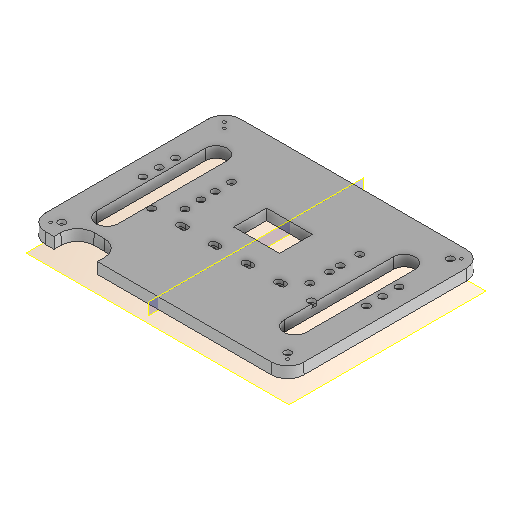
# Autodesk Inventor part: 60_Planktoscope_MicroscopeHolder_Bottom_v0
Saved by Autodesk Inventor 2024.1 (Build 281209000, 209)
## iProperties
Created: 2024-06-29
Part Number: 60_Planktoscope_MicroscopeHolder_Bottom_v0
Material: Generisch
Document SubType Name: Modeling
Designer: diederichbenedict
Density: 1 g/cm^3
Appearance: Vorgabe
Vendor: openUC2
Mass: 350.769 g
Surface Area: 894.112 cm^2
Volume: 350.769 cm^3
Author: diederichbenedict
Autodesk Inventor part; units mm, degrees
ref_plane "YZ Plane" through (0, 0, 0) normal (1, 0, 0) x (0, 1, 0)
ref_plane "XZ Plane" through (0, 0, 0) normal (0, 1, 0) x (-1, 0, 0)
ref_plane "XY Plane" through (0, 0, 0) normal (0, 0, 1) x (1, 0, 0)
ref_plane "Arbeitsebene1" through (0, -238.9229, -15) normal (0, 0, 1) x (1, 0, 0)
sketch "Skizze1" plane through (0, -238.9229, 0) normal (0, 0, 1) x (1, 0, 0)
  line L0 (-108.9123, -85.8768) -> (-108, -84.9645) construction
  line L1 (-108, -84.9645) -> (-105.5687, -87.3957) construction
  arc A0 (-105.5687, -87.3957) -> (-101.5, -88) centre (-101.5, -74) ccw construction
  line L2 (-101.5, -88) -> (-95.5, -88) construction
  line L3 (-95.5, -88) -> (-95.5, -75) construction
  arc A1 (-88.5, -68) -> (-95.5, -75) centre (-88.5, -75) ccw construction
  line L4 (-88.5, -68) -> (-62.5, -68) construction
  arc A2 (-55.5, -75) -> (-62.5, -68) centre (-62.5, -75) ccw construction
  line L5 (-55.5, -75) -> (-55.5, -88) construction
  line L6 (-55.5, -88) -> (101.7625, -88) construction
  arc A3 (101.7625, -88) -> (115.5, -74) centre (101.5, -74.0025) ccw construction
  line L7 (115.5, -74) -> (115.5, 74) construction
  arc A4 (115.5, 74) -> (101.7625, 88) centre (101.5, 74.0025) ccw construction
  line L8 (101.7625, 88) -> (-101.5, 88) construction
  arc A5 (-101.5, 88) -> (-115.5, 74) centre (-101.5, 74) ccw construction
  line L9 (-115.5, 74) -> (-115.5, -74) construction
  arc A6 (-115.5, -74) -> (-108.9123, -85.8768) centre (-101.5, -74) ccw construction
  line L10 (101.6984, -82) -> (101.3016, -82) construction
  arc A7 (101.3016, -82) -> (101.6984, -82) centre (101.5, -74.0025) ccw construction
  line L11 (95.5, 73) -> (95.5, 82) construction
  arc A8 (95.5, 73) -> (100.5, 68) centre (100.5, 73) ccw construction
  line L12 (109.5, 68) -> (100.5, 68) construction
  line L13 (109.5, 68) -> (109.5, -68) construction
  line L14 (100.5, -68) -> (109.5, -68) construction
  arc A9 (100.5, -68) -> (95.5, -73) centre (100.5, -73) ccw construction
  line L15 (95.5, -82) -> (95.5, -73) construction
  line L16 (95.5, -82) -> (-49.5, -82) construction
  line L17 (-49.5, -82) -> (-49.5, -75) construction
  arc A10 (-49.5, -75) -> (-62.5, -62) centre (-62.5, -75) ccw construction
  line L18 (-62.5, -62) -> (-88.5, -62) construction
  arc A11 (-88.5, -62) -> (-99.5163, -68.0977) centre (-88.5, -75) ccw construction
  arc A12 (-99.5163, -68.0977) -> (-100.5, -68) centre (-100.5, -73) ccw construction
  line L19 (-109.5, -68) -> (-100.5, -68) construction
  line L20 (-109.5, -68) -> (-109.5, 68) construction
  line L21 (-100.5, 68) -> (-109.5, 68) construction
  arc A13 (-100.5, 68) -> (-95.5, 73) centre (-100.5, 73) ccw construction
  line L22 (-95.5, 82) -> (-95.5, 73) construction
  line L23 (-95.5, 82) -> (95.5, 82) construction
  arc A14 (101.6984, 82) -> (101.3016, 82) centre (101.5, 74.0025) ccw construction
  line L24 (101.3016, 82) -> (101.6984, 82) construction
  line L25 (111.5331, 80.5) -> (107.9975, 76.9645) construction
  line L26 (107.9975, 76.9645) -> (104.462, 80.5) construction
  line L27 (104.462, 80.5) -> (107.9975, 84.0355) construction
  line L28 (107.9975, 84.0355) -> (111.5331, 80.5) construction
  line L29 (108, -84.0355) -> (104.4645, -80.5) construction
  line L30 (104.4645, -80.5) -> (108, -76.9645) construction
  line L31 (108, -76.9645) -> (111.5355, -80.5) construction
  line L32 (111.5355, -80.5) -> (108, -84.0355) construction
  line L33 (-108, 76.9645) -> (-111.5355, 80.5) construction
  line L34 (-111.5355, 80.5) -> (-108, 84.0355) construction
  line L35 (-108, 84.0355) -> (-104.4645, 80.5) construction
  line L36 (-104.4645, 80.5) -> (-108, 76.9645) construction
  circle A15 centre (58.5, 18.7) radius 1.4 projected
  circle A16 centre (58.5, 36.552) radius 1.4 projected
  circle A17 centre (-57.5, 20.252) radius 1.4 projected
  circle A18 centre (-57.5, 35) radius 1.4 projected
  line L37 (-60.5, 13.7) -> (-60.5, 38) construction
  line L38 (61.5, 13.7) -> (-60.5, 13.7) construction
  line L39 (61.5, 38) -> (61.5, 13.7) construction
  line L40 (61.5, 38) -> (-60.5, 38) construction
  circle A19 centre (58.5, 8.7) radius 1.4 projected
  circle A20 centre (58.5, -9.152) radius 1.4 projected
  circle A21 centre (-57.5, 7.148) radius 1.4 projected
  circle A22 centre (-57.5, -7.6) radius 1.4 projected
  line L41 (-60.5, 13.7) -> (-60.5, -10.6) construction
  line L42 (61.5, -10.6) -> (-60.5, -10.6) construction
  line L43 (61.5, -10.6) -> (61.5, 13.7) construction
  line L44 (61.5, 13.7) -> (-60.5, 13.7) construction
  line L45 (-103.5, 89.5) -> (103.5, 89.5)
  line L46 (118.5, 74.5) -> (118.5, -74.5)
  line L47 (103.5, -89.5) -> (-103.5, -89.5)
  line L48 (-118.5, -74.5) -> (-118.5, 74.5)
  arc A23 (-118.5, -74.5) -> (-103.5, -89.5) centre (-103.5, -74.5) ccw
  arc A24 (-103.5, 89.5) -> (-118.5, 74.5) centre (-103.5, 74.5) ccw
  arc A25 (118.5, 74.5) -> (103.5, 89.5) centre (103.5, 74.5) ccw
  arc A26 (103.5, -89.5) -> (118.5, -74.5) centre (103.5, -74.5) ccw
  line L49 (-95.5, -88) -> (-56.1, -88)
  line L50 (-56.1, -88) -> (-56.1, -83)
  line L51 (-71.1, -68) -> (-80.5, -68)
  line L52 (-95.5, -83) -> (-95.5, -88)
  arc A27 (-80.5, -68) -> (-95.5, -83) centre (-80.5, -83) ccw
  arc A28 (-56.1, -83) -> (-71.1, -68) centre (-71.1, -83) ccw
  line L53 (-95.5, -88) -> (-56.1, -88)
  line L54 (-56.1, -88) -> (-56.1, -89.5)
  line L55 (-56.1, -89.5) -> (-95.5, -89.5)
  line L56 (-95.5, -89.5) -> (-95.5, -88)
  point P0 (0, 238.9229)
  point P1 (-103.5567, -87.8481)
  point P2 (-95.5, -87.3481)
  point P3 (-56.1, -87.3481)
  point P4 (-56.1, -88)
  dimension "d0" = 3
  dimension "d1" = 3
  dimension "d4" = 15
  dimension "d5" = 15
  dimension "d42" = 1.5
  dimension "d43" = 1.5
  constraints: 24 end point, 13 point on circle, 12 tangent, 6 centre point, 6 parallel, 4 equal radius, 3 horizontal, 3 perpendicular, 1 point on line
  measures "d0" distance between parallel lines of L48 L9
  measures "d1" distance between parallel lines of L7 L46
  measures "d4" radius of A23
  measures "d5" radius of A27
  measures "d42" distance between parallel lines of L47 L49
  measures "d43" distance between parallel lines of L45 L8
extrude "Extrusion1" add sketch "Skizze1" along normal blind 10 draft -1 contours L45 A25 L46 A26 L47 L54 L50 A28 L51 A27 L52 L56 A23 L48 A24
sketch "Skizze3" plane through (0, -238.9229, 10) normal (0, 0, 1) x (1, 0, 0)
  line L0 (118.3254, 74.5) -> (118.3254, -74.5) projected
  arc A0 (118.3254, 74.5) -> (103.5, 89.3254) centre (103.5, 74.5) ccw projected
  line L1 (-103.5, 89.3254) -> (103.5, 89.3254) projected
  arc A1 (-103.5, 89.3254) -> (-118.3254, 74.5) centre (-103.5, 74.5) ccw projected
  line L2 (-118.3254, -74.5) -> (-118.3254, 74.5) projected
  arc A2 (-118.3254, -74.5) -> (-103.5, -89.3254) centre (-103.5, -74.5) ccw projected
  line L3 (-95.6746, -89.3254) -> (-103.5, -89.3254) projected
  line L4 (-95.6746, -83) -> (-95.6746, -89.3254) projected
  arc A3 (-80.5, -67.8254) -> (-95.6746, -83) centre (-80.5, -83) ccw projected
  line L5 (-71.1, -67.8254) -> (-80.5, -67.8254) projected
  arc A4 (-55.9254, -83) -> (-71.1, -67.8254) centre (-71.1, -83) ccw projected
  line L6 (-55.9254, -89.3254) -> (-55.9254, -83) projected
  arc A5 (103.5, -89.3254) -> (118.3254, -74.5) centre (103.5, -74.5) ccw projected
  circle A6 centre (58.5, 18.7) radius 1.5746 projected
  circle A7 centre (58.5, 36.552) radius 1.5746 projected
  circle A8 centre (-57.5, 20.252) radius 1.5746 projected
  circle A9 centre (-57.5, 35) radius 1.5746 projected
  circle A10 centre (58.5, 8.7) radius 1.5746 projected
  circle A11 centre (58.5, -9.152) radius 1.5746 projected
  circle A12 centre (-57.5, 7.148) radius 1.5746 projected
  circle A13 centre (-57.5, -7.6) radius 1.5746 projected
  line L7 (103.5, -89.3254) -> (-55.9254, -89.3254) projected
  line L8 (103.5, -74.5) -> (-103.5, -74.5)
  line L9 (-103.5, -74.5) -> (-103.5, 74.5)
  line L10 (-103.5, 74.5) -> (103.5, 74.5)
  line L11 (103.5, 74.5) -> (103.5, -74.5)
  line L12 (-108.5, -79.5) -> (108.5, -79.5)
  line L13 (108.5, -79.5) -> (108.5, 79.5)
  line L14 (108.5, 79.5) -> (-108.5, 79.5)
  line L15 (-108.5, 79.5) -> (-108.5, -79.5)
  point P0 (0, 238.9229)
  dimension "d56" = 5
  constraints: 16 end point, 4 parallel, 2 perpendicular, 1 horizontal, 3 other
  measures "d56" distance between parallel lines of L8 L12
hole "Bohrung1" at (-103.5, -164.4229, 10) at (-103.5, -313.4229, 10) at (103.5, -313.4229, 10) at (103.5, -164.4229, 10) at (108.5, -159.4229, 10) at (108.5, -318.4229, 10) at (-108.5, -159.4229, 10) at (-108.5, -318.4229, 10) direction (0, 0, -1) diameter 2.8 end through all
sketch "Skizze4" plane through (0, -238.9229, 10) normal (0, 0, 1) x (1, 0, 0)
  line L0 (-2.75, 38) -> (-2.75, 23.7) projected
  line L1 (-6.0553, 13.7) -> (-6.0553, 30)
  line L2 (20.9, 30.6837) -> (20.9, 6.6837) projected
  line L3 (20.9, 30.6837) -> (-20.9567, 30.6837)
  line L4 (-20.9567, 30.6837) -> (-20.9567, 0.5738)
  line L5 (-20.9567, 0.5738) -> (20.9, 0.5738)
  line L6 (20.9, 0.5738) -> (20.9, 30.6837)
  circle A0 centre (-57.5, 7.148) radius 1.4 projected
  circle A1 centre (-57.5, -10.7039) radius 1.4 projected
  circle A2 centre (58.5, 5.5961) radius 1.4 projected
  circle A3 centre (58.5, -9.152) radius 1.4 projected
  line L7 (-1.5, 2.2357) -> (-1.5, 12.148) projected
  line L8 (-19.5, 2.2357) -> (-1.5, 2.2357) projected
  line L9 (-19.5, 12.148) -> (-19.5, 2.2357) projected
  line L10 (-19.5, 12.148) -> (-60.5, 12.148) projected
  line L11 (-60.5, 12.148) -> (-60.5, -12.152) projected
  line L12 (61.5, -12.152) -> (-60.5, -12.152) projected
  line L13 (61.5, -12.152) -> (61.5, 12.148) projected
  line L14 (61.5, 12.148) -> (-1.5, 12.148) projected
  point P0 (0, 238.9229)
  constraints: 10 end point, 2 parallel, 1 horizontal, 1 perpendicular, 1 vertical, 2 other
extrude "Extrusion3" cut sketch "Skizze4" against normal through all contours L2 L14 L7 L8 L9 L10 L4 L3 | L2 L6 L5 L4 L10 L9 L8 L7 L14
sketch "Skizze5" plane through (0, -238.9229, 10) normal (0, 0, 1) x (1, 0, 0)
  line L0 (-20.9567, 30.6837) -> (20.9, 30.6837) projected
  line L1 (20.9, 30.6837) -> (20.9, 0.5738) projected
  line L2 (20.9, 0.5738) -> (-20.9567, 0.5738) projected
  line L3 (-20.9567, 0.5738) -> (-20.9567, 30.6837) projected
  circle A0 centre (103.5, 74.5) radius 1.4 projected
  circle A1 centre (103.5, -74.5) radius 1.4 projected
  circle A2 centre (-103.5, -74.5) radius 1.4 projected
  circle A3 centre (-103.5, 74.5) radius 1.4 projected
  line L4 (118.3254, 74.5) -> (118.3254, -74.5) projected
  arc A4 (118.3254, 74.5) -> (103.5, 89.3254) centre (103.5, 74.5) ccw projected
  line L5 (-103.5, 89.3254) -> (103.5, 89.3254) projected
  arc A5 (-103.5, 89.3254) -> (-118.3254, 74.5) centre (-103.5, 74.5) ccw projected
  line L6 (-118.3254, -74.5) -> (-118.3254, 74.5) projected
  arc A6 (-118.3254, -74.5) -> (-103.5, -89.3254) centre (-103.5, -74.5) ccw projected
  line L7 (-95.6746, -89.3254) -> (-103.5, -89.3254) projected
  line L8 (-95.6746, -83) -> (-95.6746, -89.3254) projected
  arc A7 (-80.5, -67.8254) -> (-95.6746, -83) centre (-80.5, -83) ccw projected
  line L9 (-71.1, -67.8254) -> (-80.5, -67.8254) projected
  arc A8 (-55.9254, -83) -> (-71.1, -67.8254) centre (-71.1, -83) ccw projected
  line L10 (-55.9254, -89.3254) -> (-55.9254, -83) projected
  arc A9 (103.5, -89.3254) -> (118.3254, -74.5) centre (103.5, -74.5) ccw projected
  circle A10 centre (58.5, 18.7) radius 1.5746 projected
  circle A11 centre (58.5, 36.552) radius 1.5746 projected
  circle A12 centre (-57.5, 20.252) radius 1.5746 projected
  circle A13 centre (-57.5, 35) radius 1.5746 projected
  circle A14 centre (58.5, 8.7) radius 1.5746 projected
  circle A15 centre (58.5, -9.152) radius 1.5746 projected
  circle A16 centre (-57.5, 7.148) radius 1.5746 projected
  circle A17 centre (-57.5, -7.6) radius 1.5746 projected
  line L11 (-73.1917, -22.4328) -> (70.9104, -22.4328)
  line L12 (102.338, 36.5746) -> (102.338, -9.1746)
  line L13 (103.5, -89.3254) -> (-55.9254, -89.3254) projected
  point P0 (0, 238.9229)
  point P1 (-43.1917, -22.4328)
  point P2 (-13.1917, -22.4328)
  point P3 (16.8083, -22.4328)
  point P4 (46.8083, -22.4328)
  point P5 (102.338, 13.7)
  point P6 (102.338, -1.3)
  point P7 (102.338, 28.7)
  point P8 (102.338, 13.7)
  dimension "d21" = 30
  dimension "d36" = 15
  dimension "d39" = 15
  constraints: 4 end point, 3 vertical, 2 horizontal, 1 coincident, 1 midpoint, 7 other
  measures "d21" distance of point (-73.192, -22.433) point (-43.192, -22.433)
  measures "d36" distance of point (102.338, 13.7) point (102.338, -1.3)
  measures "d39" distance of point (102.338, 13.7) point (102.338, 28.7)
hole "Bohrung2" at (-73.1917, -261.3557, 10) at (-43.1917, -261.3557, 10) at (-13.1917, -261.3557, 10) at (16.8083, -261.3557, 10) at (46.8083, -261.3557, 10) at (102.338, -240.2229, 10) at (102.338, -225.2229, 10) at (102.338, -210.2229, 10) direction (0, 0, -1) diameter 2.8 end through all
ref_plane "Arbeitsebene2" through (0, -313.4229, 6788.8605) normal (-1, 0, 0) x (0, -1, 0)
mirror "Spiegeln1" about plane through (0, -313.4229, 6788.8605) normal (-1, 0, 0) of "Bohrung2", "Extrusion3", "Bohrung1"
sketch "Skizze6" plane through (0, -238.9229, 10) normal (0, 0, 1) x (1, 0, 0)
  line L0 (20.9567, 0.5738) -> (-20.9567, 0.5738) projected
  line L1 (-20.9567, 0.5738) -> (-20.9567, 30.6837) projected
  line L2 (-20.9567, 30.6837) -> (20.9567, 30.6837) projected
  line L3 (20.9567, 30.6837) -> (20.9567, 0.5738) projected
  circle A0 centre (-102.338, 13.7) radius 1.4 projected
  circle A1 centre (-102.338, -1.3) radius 1.4 projected
  circle A2 centre (-46.8083, -22.4328) radius 1.4 projected
  circle A3 centre (-16.8083, -22.4328) radius 1.4 projected
  circle A4 centre (13.1917, -22.4328) radius 1.4 projected
  circle A5 centre (43.1917, -22.4328) radius 1.4 projected
  circle A6 centre (73.1917, -22.4328) radius 1.4 projected
  circle A7 centre (-102.338, 28.7) radius 1.4 projected
  circle A8 centre (102.338, 28.7) radius 1.4 projected
  circle A9 centre (102.338, 13.7) radius 1.4 projected
  circle A10 centre (102.338, -1.3) radius 1.4 projected
  circle A11 centre (46.8083, -22.4328) radius 1.4 projected
  circle A12 centre (16.8083, -22.4328) radius 1.4 projected
  circle A13 centre (-13.1917, -22.4328) radius 1.4 projected
  circle A14 centre (-43.1917, -22.4328) radius 1.4 projected
  circle A15 centre (-73.1917, -22.4328) radius 1.4 projected
  circle A16 centre (103.5, 74.5) radius 1.4 projected
  circle A17 centre (103.5, -74.5) radius 1.4 projected
  circle A18 centre (-103.5, -74.5) radius 1.4 projected
  circle A19 centre (-103.5, 74.5) radius 1.4 projected
  circle A20 centre (-57.5, -7.6) radius 1.5746 projected
  circle A21 centre (-57.5, 7.148) radius 1.5746 projected
  circle A22 centre (58.5, -9.152) radius 1.5746 projected
  circle A23 centre (58.5, 8.7) radius 1.5746 projected
  circle A24 centre (-57.5, 35) radius 1.5746 projected
  circle A25 centre (-57.5, 20.252) radius 1.5746 projected
  circle A26 centre (58.5, 36.552) radius 1.5746 projected
  circle A27 centre (58.5, 18.7) radius 1.5746 projected
  line L4 (118.3254, 74.5) -> (118.3254, -74.5) projected
  arc A28 (118.3254, 74.5) -> (103.5, 89.3254) centre (103.5, 74.5) ccw projected
  line L5 (-103.5, 89.3254) -> (103.5, 89.3254) projected
  arc A29 (-103.5, 89.3254) -> (-118.3254, 74.5) centre (-103.5, 74.5) ccw projected
  line L6 (-118.3254, -74.5) -> (-118.3254, 74.5) projected
  arc A30 (-118.3254, -74.5) -> (-103.5, -89.3254) centre (-103.5, -74.5) ccw projected
  line L7 (-95.6746, -89.3254) -> (-103.5, -89.3254) projected
  line L8 (-95.6746, -83) -> (-95.6746, -89.3254) projected
  arc A31 (-80.5, -67.8254) -> (-95.6746, -83) centre (-80.5, -83) ccw projected
  line L9 (-71.1, -67.8254) -> (-80.5, -67.8254) projected
  arc A32 (-55.9254, -83) -> (-71.1, -67.8254) centre (-71.1, -83) ccw projected
  line L10 (-55.9254, -89.3254) -> (-55.9254, -83) projected
  line L11 (103.5, -89.3254) -> (-55.9254, -89.3254) projected
  arc A33 (103.5, -89.3254) -> (118.3254, -74.5) centre (103.5, -74.5) ccw projected
  line L12 (85.8131, 50) -> (85.8131, -50) construction
  line L13 (75.8131, 50) -> (75.8131, -50)
  line L14 (95.8131, -50) -> (95.8131, 50)
  arc A34 (95.8131, 50) -> (75.8131, 50) centre (85.8131, 50) ccw
  arc A35 (75.8131, -50) -> (95.8131, -50) centre (85.8131, -50) ccw
  line L15 (-86.5043, 50) -> (-86.5043, -50) construction
  line L16 (-96.5043, 50) -> (-96.5043, -50)
  line L17 (-76.5043, -50) -> (-76.5043, 50)
  arc A36 (-76.5043, 50) -> (-96.5043, 50) centre (-86.5043, 50) ccw
  arc A37 (-96.5043, -50) -> (-76.5043, -50) centre (-86.5043, -50) ccw
  point P0 (0, 238.9229)
  point P1 (85.8131, 0)
  point P2 (-86.5043, 0)
  dimension "d44" = 50
  dimension "d45" = 20
  dimension "d46" = 20
  constraints: 16 end point, 8 point on circle, 8 tangent, 4 centre point, 3 parallel, 2 midpoint, 1 vertical
  measures "d44" distance of point (85.813, 0) L12.end
  measures "d45" diameter of A35
  measures "d46" diameter of A37
extrude "Extrusion4" cut sketch "Skizze6" against normal through all contours A34 L14 A35 L13 | A36 L17 A37 L16
sketch "Skizze7" plane through (0, -238.9229, 10) normal (0, 0, 1) x (1, 0, 0)
  line L0 (-76.5043, 50) -> (-76.5043, -50) projected
  arc A0 (-96.5043, -50) -> (-76.5043, -50) centre (-86.5043, -50) ccw projected
  line L1 (-96.5043, -50) -> (-96.5043, 50) projected
  arc A1 (-76.5043, 50) -> (-96.5043, 50) centre (-86.5043, 50) ccw projected
  line L2 (95.8131, 50) -> (95.8131, -50) projected
  arc A2 (75.8131, -50) -> (95.8131, -50) centre (85.8131, -50) ccw projected
  line L3 (75.8131, -50) -> (75.8131, 50) projected
  arc A3 (95.8131, 50) -> (75.8131, 50) centre (85.8131, 50) ccw projected
  line L4 (20.9567, 0.5738) -> (-20.9567, 0.5738) projected
  line L5 (-20.9567, 0.5738) -> (-20.9567, 30.6837) projected
  line L6 (-20.9567, 30.6837) -> (20.9567, 30.6837) projected
  line L7 (20.9567, 30.6837) -> (20.9567, 0.5738) projected
  circle A4 centre (-102.338, 13.7) radius 1.4 projected
  circle A5 centre (-102.338, -1.3) radius 1.4 projected
  circle A6 centre (-46.8083, -22.4328) radius 1.4 projected
  circle A7 centre (-16.8083, -22.4328) radius 1.4 projected
  circle A8 centre (13.1917, -22.4328) radius 1.4 projected
  circle A9 centre (43.1917, -22.4328) radius 1.4 projected
  circle A10 centre (73.1917, -22.4328) radius 1.4 projected
  circle A11 centre (-102.338, 28.7) radius 1.4 projected
  circle A12 centre (102.338, 28.7) radius 1.4 projected
  circle A13 centre (102.338, 13.7) radius 1.4 projected
  circle A14 centre (102.338, -1.3) radius 1.4 projected
  circle A15 centre (46.8083, -22.4328) radius 1.4 projected
  circle A16 centre (16.8083, -22.4328) radius 1.4 projected
  circle A17 centre (-13.1917, -22.4328) radius 1.4 projected
  circle A18 centre (-43.1917, -22.4328) radius 1.4 projected
  circle A19 centre (-73.1917, -22.4328) radius 1.4 projected
  circle A20 centre (103.5, 74.5) radius 1.4 projected
  circle A21 centre (103.5, -74.5) radius 1.4 projected
  circle A22 centre (-103.5, -74.5) radius 1.4 projected
  circle A23 centre (-103.5, 74.5) radius 1.4 projected
  circle A24 centre (-57.5, -7.6) radius 1.5746 projected
  circle A25 centre (-57.5, 7.148) radius 1.5746 projected
  circle A26 centre (58.5, -9.152) radius 1.5746 projected
  circle A27 centre (58.5, 8.7) radius 1.5746 projected
  circle A28 centre (-57.5, 35) radius 1.5746 projected
  circle A29 centre (-57.5, 20.252) radius 1.5746 projected
  circle A30 centre (58.5, 36.552) radius 1.5746 projected
  circle A31 centre (58.5, 18.7) radius 1.5746 projected
  line L8 (118.3254, 74.5) -> (118.3254, -74.5) projected
  arc A32 (118.3254, 74.5) -> (103.5, 89.3254) centre (103.5, 74.5) ccw projected
  line L9 (-103.5, 89.3254) -> (103.5, 89.3254) projected
  arc A33 (-103.5, 89.3254) -> (-118.3254, 74.5) centre (-103.5, 74.5) ccw projected
  line L10 (-118.3254, -74.5) -> (-118.3254, 74.5) projected
  arc A34 (-118.3254, -74.5) -> (-103.5, -89.3254) centre (-103.5, -74.5) ccw projected
  line L11 (-95.6746, -89.3254) -> (-103.5, -89.3254) projected
  line L12 (-95.6746, -83) -> (-95.6746, -89.3254) projected
  arc A35 (-80.5, -67.8254) -> (-95.6746, -83) centre (-80.5, -83) ccw projected
  line L13 (-71.1, -67.8254) -> (-80.5, -67.8254) projected
  arc A36 (-55.9254, -83) -> (-71.1, -67.8254) centre (-71.1, -83) ccw projected
  line L14 (-55.9254, -89.3254) -> (-55.9254, -83) projected
  line L15 (103.5, -89.3254) -> (-55.9254, -89.3254) projected
  arc A37 (103.5, -89.3254) -> (118.3254, -74.5) centre (103.5, -74.5) ccw projected
  point P0 (0, 238.9229)
hole "Bohrung3" at (102.338, -210.2229, 10) at (102.338, -225.2229, 10) at (102.338, -240.2229, 10) at (73.1917, -261.3557, 10) at (46.8083, -261.3557, 10) at (43.1917, -261.3557, 10) at (16.8083, -261.3557, 10) at (13.1917, -261.3557, 10) at (-13.1917, -261.3557, 10) at (-16.8083, -261.3557, 10) at (-43.1917, -261.3557, 10) at (-46.8083, -261.3557, 10) at (-57.5, -246.5229, 10) at (-57.5, -231.7749, 10) at (-57.5, -218.671, 10) at (-57.5, -203.9229, 10) at (-73.1917, -261.3557, 10) at (-103.5, -313.4229, 10) at (-102.338, -240.2229, 10) at (-102.338, -225.2229, 10) at (-102.338, -210.2229, 10) at (103.5, -313.4229, 10) at (103.5, -164.4229, 10) at (58.5, -248.0749, 10) at (58.5, -230.2229, 10) at (58.5, -220.2229, 10) at (58.5, -202.371, 10) direction (0, 0, -1) diameter 2.8 depth 8 tip angle 150 counterbore diameter 6.5 counterbore depth 3.5
